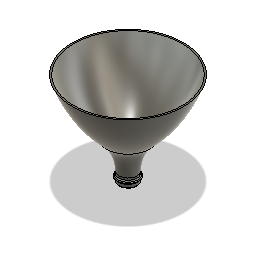
Fill funnel v3 (Autodesk Fusion 360 design; units mm, degrees)
Autodesk Fusion 360 part; units mm, degrees
sketch "Sketch1" plane through (0, 0, 0) normal (0, 0, 1) x (1, 0, 0)
  line L0 (9.925, 8.0443) -> (9.925, 10.1613)
  arc A0 (23.2698, 41.8312) -> (9.925, 10.1613) centre (54.177, 10.1613) ccw
  arc A1 (23.2698, 41.8312) -> (60, 100) centre (-80.1817, 147.8356) ccw
  line L1 (23.2698, 41.8312) -> (0, 19.1218) construction
  line L2 (0, 0) -> (0, 100)
  line L3 (8.325, 0) -> (8.325, 10.1613)
  arc A2 (22.1523, 42.9762) -> (8.325, 10.1613) centre (54.177, 10.1613) ccw
  arc A3 (22.1523, 42.9762) -> (58.3083, 100) centre (-80.1817, 147.8356) ccw
  line L4 (8.325, 0) -> (8.8407, 0)
  line L5 (60, 100) -> (58.3083, 100)
  line L6 (9.1943, 0.1464) -> (9.5791, 0.5313)
  line L7 (9.925, 5) -> (10.925, 5)
  line L8 (11.425, 5.5) -> (11.425, 5.5087)
  line L9 (11.2786, 5.8623) -> (10.5108, 6.6301)
  arc A4 (9.925, 8.0443) -> (10.5108, 6.6301) centre (11.925, 8.0443) ccw
  line L10 (9.925, 5) -> (9.725, 0.8607)
  arc A5 (11.425, 5.5087) -> (11.2786, 5.8623) centre (10.925, 5.5087) ccw
  arc A6 (10.925, 5) -> (11.425, 5.5) centre (10.925, 5.5) ccw
  arc A7 (8.8407, 0) -> (9.1943, 0.1464) centre (8.8407, 0.5) ccw
  arc A8 (9.5791, 0.5313) -> (9.725, 0.8607) centre (9.2256, 0.8849) ccw
  point P0 (11.425, 5)
  dimension "d1" = 100
  dimension "d2" = 120
  dimension "d3" = 45.698
  dimension "d4" = 19.85
  dimension "d7" = 45
  dimension "d8" = 1.5
  dimension "d9" = 5
  dimension "d10" = 3.1
  dimension "d11" = 2
  dimension "d12" = 45
  dimension "d13" = 0.5
  dimension "d14" = 0.5
  dimension "d15" = 0.5
  dimension "d17" = 0.2
  constraint vertical L0
  constraint tangent L0 A0
  constraint tangent A0 A1
  constraint tangent A0 L1
  constraint coincident L2.start origin
  constraint vertical L2
  constraint coincident L1.end L2
  constraint horizontal A1.end L2.end
  constraint perpendicular L0 L4
  constraint perpendicular L0 L5
  constraint concentric A0 A2
  constraint concentric A1 A3
  constraint tangent L3 A2
  constraint tangent A2 A3
  constraint horizontal L2.start L3.start
  constraint coincident L0 L7.start
  constraint perpendicular L0 L7
  constraint perpendicular L7 L8
  constraint tangent L0 A4
  constraint tangent L9 A4
  constraint tangent L8 A5
  constraint tangent L9 A5
  constraint coincident P0 L7
  constraint coincident P0 L8
  constraint tangent L7 A6
  constraint tangent L8 A6
  constraint tangent L6 A7
  constraint tangent L4 A7
  constraint tangent L6 A8
  constraint tangent L10 A8
  constraint equal A7 A8
  measures "d1" distance of L2.start L2.end
  measures "d3" angle of L1 L2
  measures "d7" angle of L0 L6
  measures "d8" distance of L7.start P0
  measures "d9" distance of L4 L7
  measures "d10" distance of L3 L8
  measures "d11" radius of A4
  measures "d12" angle of L8 L9
  measures "d13" radius of A5
  measures "d14" radius of A6
  measures "d15" radius of A7
  measures "d17" horizontal distance of L7.start L10.end
revolve "Revolve1" add sketch "Sketch1" angle 360 about axis through (0, 0, 0) along (0, 1, 0)
equation "d4 = 20 mm - 0.15 mm"
